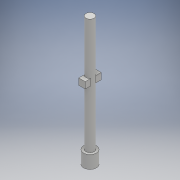
# Autodesk Inventor part: Rotation
Saved by Autodesk Inventor 2018 (Build 220112000, 112)
## iProperties
Created: 2019-07-18
Part Number: Rotation
Material: Generic
Document SubType Name: Modeling
Designer: aal_9
Density: 1 g/cm^3
Appearance: Default
Author: aal_9
Autodesk Inventor part; units mm, degrees
ref_plane "YZ Plane" through (0, 0, 0) normal (1, 0, 0) x (0, 1, 0)
sketch "Sketch1" plane through (0, 0, 0) normal (0, 0, 1) x (1, 0, 0)
  circle A0 centre (0, 0) radius 3.2
  dimension "d0" = 6.4
  constraints: 1 centre point, 1 coincident
  measures "d0" diameter of A0
extrude "Extrusion1" add sketch "Sketch1" along normal blind 90
ref_plane "Work Plane2" through (0, 3.2, 0) normal (0, 1, 0) x (-1, 0, 0)
sketch "Sketch7" plane through (0, 3.2, 0) normal (0, 1, 0) x (-1, 0, 0)
  line L0 (2.5, 50) -> (-2.5, 50)
  line L1 (-2.5, 50) -> (-2.5, 45)
  line L2 (-2.5, 45) -> (2.5, 45)
  line L3 (2.5, 45) -> (2.5, 50)
  line L4 (-3.2, 0) -> (3.2, 0) projected
  line L5 (3.2, 90) -> (-3.2, 90) projected
  point P0 (0, 0)
  dimension "d30" = 5
  dimension "d31" = 5
  dimension "d32" = 2.5
  dimension "d42" = 40
  constraints: 8 end point, 2 parallel, 1 horizontal, 1 perpendicular
  measures "d30" distance of L0.start L0.end
  measures "d31" distance of L2.end L0.start
  measures "d32" distance from line of point (0, 0) L3
  measures "d42" distance between parallel lines of L5 L0
extrude "Extrusion6" add sketch "Sketch7" against normal blind 9.4 and the other way blind 3
sketch "Sketch9" plane through (0, 0, 0) normal (0, 0, -1) x (-1, 0, 0)
  circle A0 centre (0, 0) radius 5
  dimension "d43" = 10
  constraints: 1 centre point, 1 coincident
  measures "d43" diameter of A0
extrude "Extrusion8" add sketch "Sketch9" along normal blind 10
sketch "Sketch10" plane through (0, 0, -10) normal (0, 0, -1) x (-1, 0, 0)
  arc A0 (-2.8284, 1) -> (2.8284, 1) centre (0, 0) ccw
  line L0 (-2.8284, 1) -> (2.8284, 1)
  dimension "d46" = 6
  dimension "d47" = 1
  constraints: 2 end point, 2 point on circle, 1 centre point, 1 coincident, 1 horizontal
  measures "d46" diameter of A0
  measures "d47" distance from line of point (0, 0) L0
extrude "Extrusion9" cut sketch "Sketch10" against normal blind 7
ref_plane "Work Plane4" through (0, 5, 0) normal (0, 1, 0) x (-1, 0, 0)
sketch "Sketch12" plane through (0, 5, 0) normal (0, 1, 0) x (-1, 0, 0)
  circle A0 centre (0, -6.5) radius 0.8
  line L0 (-5, -10) -> (5, -10) projected
  point P0 (0, 0)
  dimension "d54" = 1.6
  dimension "d55" = 3.5
  constraints: 1 centre point
  measures "d54" diameter of A0
  measures "d55" distance from line of L0 A0.centre
extrude "Extrusion11" cut sketch "Sketch12" against normal up to next
equation "\"d32\" = 0.5 * d30"
body "Solid1"
